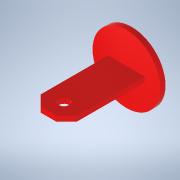
# Autodesk Inventor part: Deckel
Saved by Autodesk Inventor 2022 (Build 260153000, 153)
## iProperties
Created: 2022-06-01
Part Number: Deckel
Material: Generisch
Document SubType Name: Modeling
Designer: kaebi
Density: 1 g/cm^3
Appearance: Glatt - Rot
Author: kaebi
Autodesk Inventor part; units mm, degrees
ref_plane "YZ Plane" through (0, 0, 0) normal (1, 0, 0) x (0, 1, 0)
ref_plane "XZ Plane" through (0, 0, 0) normal (0, 1, 0) x (-1, 0, 0)
ref_plane "XY Plane" through (0, 0, 0) normal (0, 0, 1) x (1, 0, 0)
sketch "Skizze1" plane through (0, 0, 0) normal (0, 0, 1) x (1, 0, 0)
  circle A0 centre (0, 0) radius 6.5
  dimension "d11" = 13
  constraints: 1 centre point, 1 coincident
  measures "d11" diameter of A0
extrude "Extrusion1" add sketch "Skizze1" along normal blind 1
sketch "Skizze2" plane through (0, 0, 0) normal (0, 1, 0) x (-1, 0, 0)
  line L0 (6.5, 1) -> (-6.5, 1) projected
  line L1 (3.5, 1) -> (-3.5, 1)
  line L2 (-3.5, 1) -> (-3.5, 16)
  line L3 (-3.5, 16) -> (3.5, 16)
  line L4 (3.5, 16) -> (3.5, 1)
  line L5 (0, -1) -> (0, 20) projected
  circle A0 centre (0, 13) radius 1
  point P0 (-3.5, 1)
  dimension "d2" = 15
  dimension "d3" = 7
  dimension "d4" = 2
  dimension "d5" = 3
  constraints: 8 end point, 2 parallel, 2 point on line, 1 centre point, 1 horizontal, 1 perpendicular, 1 other
  measures "d2" distance of L3.end L1.start
  measures "d3" distance of L2.end L3.end
  measures "d4" diameter of A0
  measures "d5" distance from line of A0.centre L3
extrude "Extrusion2" add sketch "Skizze2" along normal mid plane 1 contours L0 L5 A0 L3 L4 | L0 L2 L3 L5 A0
chamfer "Fase1" distance 2 angle 45 2 edges at (3.5, 0, 16) (-3.5, 0, 16)
